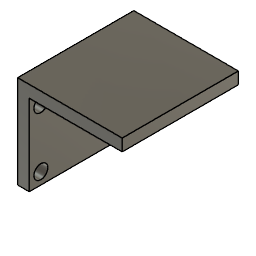
L shape (Autodesk Fusion 360 design; units mm, degrees)
Autodesk Fusion 360 part; units mm, degrees
sketch "Sketch1" plane through (0, 0, 0) normal (0, 1, 0) x (1, 0, 0)
  line L0 (-39.9507, -29.6666) -> (-39.6666, -29.6666)
  line L1 (-39.9507, -29.6666) -> (-39.9507, 40)
  line L2 (-39.9507, 40) -> (-50, 40)
  line L3 (-50, 40) -> (-50, -29.6666)
  line L4 (-39.9507, -29.6666) -> (40, -29.6666)
  line L5 (40, -29.6666) -> (40, -40)
  line L6 (40, -40) -> (-39.9507, -40)
  line L7 (-50, -40) -> (-50, -29.6666)
  line L8 (-50, -40) -> (-39.9507, -40)
  constraint horizontal L0
  constraint vertical L1
  constraint horizontal L2
  constraint vertical L3
  constraint horizontal L4
  constraint vertical L5
  constraint horizontal L6
  constraint vertical L7
  constraint perpendicular L1 L8
extrude "Extrude1" add sketch "Sketch1" along normal blind 100
sketch "Sketch2" plane through (-39.9507, 0, 0) normal (1, 0, 0) x (0, 1, 0)
  line L0 (0, 29.6666) -> (0, -40)
  line L1 (0, -40) -> (100, -40)
  line L2 (100, -40) -> (100, 29.6666)
  line L3 (100, 29.6666) -> (0, 29.6666)
  circle A0 centre (10, 20) radius 6
  circle A1 centre (90, 20) radius 6
  circle A2 centre (10, -30) radius 6
  circle A3 centre (90, -30) radius 6
  dimension "d3" = 12
  dimension "d6" = 80
  dimension "d7" = -50
  measures "d3" diameter of A0
extrude "Extrude2" cut sketch "Sketch2" against normal up to surface (10.0493 mm away) contours A0 | A1 | A2 | A3
